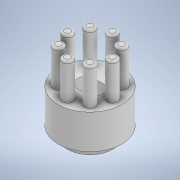
# Autodesk Inventor part: TT motor  attach to linear motion gear adapter
Saved by Autodesk Inventor 2022 (Build 260153000, 153)
## iProperties
Created: 2021-10-31
Part Number: TT motor  attach to linear motion gear adapter
Material: Generic
Document SubType Name: Modeling
Designer: alecw
Density: 1 g/cm^3
Appearance: Default
Author: alecw
Autodesk Inventor part; units mm, degrees
ref_plane "YZ Plane" through (0, 0, 0) normal (1, 0, 0) x (0, 1, 0)
ref_plane "XZ Plane" through (0, 0, 0) normal (0, 1, 0) x (-1, 0, 0)
ref_plane "XY Plane" through (0, 0, 0) normal (0, 0, 1) x (1, 0, 0)
sketch "Sketch1" plane through (0, 0, 0) normal (0, 1, 0) x (-1, 0, 0)
  circle A0 centre (0, 0) radius 2.5
  line L0 (0, 0) -> (0, 4.9)
  circle A1 centre (0, 4.9) radius 1.15
  circle A2 centre (0, 0) radius 2.7
  line L1 (0, 0) -> (0, 1.9)
  line L2 (0, 0) -> (0, -1.9)
  line L3 (0, 1.9) -> (-1.9183, 1.9)
  line L4 (0, -1.9) -> (-1.9183, -1.9)
  line L5 (0, -1.9) -> (1.9183, -1.9)
  line L6 (0, 1.9) -> (1.9183, 1.9)
  circle A3 centre (0, 0) radius 7
  circle A4 centre (-3.4648, 3.4648) radius 1.15
  circle A5 centre (-4.9, 0) radius 1.15
  circle A6 centre (-3.4648, -3.4648) radius 1.15
  circle A7 centre (0, -4.9) radius 1.15
  circle A8 centre (3.4648, -3.4648) radius 1.15
  circle A9 centre (4.9, 0) radius 1.15
  circle A10 centre (3.4648, 3.4648) radius 1.15
  circle A11 centre (0, 0) radius 4.9
  circle A12 centre (0, 0) radius 2.8
  line L7 (1.9183, -1.9) -> (2.0567, -1.9)
  line L8 (1.9183, 1.9) -> (2.0567, 1.9)
  line L9 (-1.9183, 1.9) -> (-2.0567, 1.9)
  line L10 (-1.9183, -1.9) -> (-2.0567, -1.9)
  point P0 (-1.6248, 1.9)
  point P1 (1.6248, 1.9)
  point P2 (1.6248, -1.9)
  point P3 (-1.6248, -1.9)
  dimension "d0" = 5
  dimension "d1" = 4.9
  dimension "d2" = 2.3
  dimension "d3" = 5.4
  dimension "d4" = 1.9
  dimension "d5" = 1.9
  dimension "d6" = 14
  dimension "d9" = 360
  dimension "d26" = 5.6
  constraints: 22 end point, 12 centre point, 8 point on circle, 6 coincident, 6 point on line, 2 horizontal, 2 parallel, 1 horizontal alignment, 1 vertical, 19 other
  measures "d0" diameter of A0
  measures "d1" distance of L0.start L0.end
  measures "d2" diameter of A1
  measures "d3" diameter of A2
  measures "d4" distance of L1.start L1.end
  measures "d5" distance of L1.start L2.end
  measures "d6" diameter of A3
  measures "d26" diameter of A12
extrude "Extrusion1" add sketch "Sketch1" along normal blind 3 contours A1 A11 L0 | A1 A11 A10 A9 A8 A7 A6 A5 A4 | L0 A11 A1 | A11 A1 | A11 A4 | A4 A11 | A11 A10 | A10 A11 | A11 A5 | A5 A11 | A11 A9 | A9 A11 | A11 A6 | A6 A11 | A11 A8 | A8 A11 | A11 A7 | A7 A11 | A3
extrude "Extrusion2" add sketch "Sketch1" along normal blind 6.5 from surface at 3 contours L6 L0 A0 | A0 L0 A2 L6 | L5 A2 L4 A0 | A0 L4 L5 | L0 L3 A0 | A0 L3 A2 L0 | A2 L0 A12 L8 | L7 A12 L10 A2 | A2 L9 A12 L0 | A1 A11 L0 | A1 A11 A10 A9 A8 A7 A6 A5 A4 | L0 A11 A1 | A11 A1 | A11 A4 | A4 A11 | A11 A10 | A10 A11 | A11 A5 | A5 A11 | A11 A9 | A9 A11 | A11 A6 | A6 A11 | A11 A8 | A8 A11 | A11 A7 | A7 A11 | A3
extrude "Extrusion3" add sketch "Sketch1" along normal blind 8 from surface at 9.5 contours A1 A11 L0 | L0 A11 A1 | A11 A1 | A11 A4 | A4 A11 | A11 A10 | A10 A11 | A11 A5 | A5 A11 | A11 A9 | A9 A11 | A11 A6 | A6 A11 | A11 A8 | A8 A11 | A11 A7 | A7 A11
fillet "Fillet1" radius 0.5 8 edges at (-3.75, 17.5, 0) (-2.3148, 17.5, -3.4648) (1.15, 17.5, -4.9) (4.6148, 17.5, -3.4648) (4.6148, 17.5, 3.4648) (6.05, 17.5, 0) (1.15, 17.5, 4.9) (-2.3148, 17.5, 3.4648)
chamfer "Chamfer1" distance 2 angle 45 1 edges at (7, 0, 0)
extrude "Extrusion4" add sketch "Sketch1" against normal blind 1 from surface at 3 contours L6 L0 A0 | A0 L0 A2 L6 | L5 A2 L4 A0 | A0 L4 L5 | L0 L3 A0 | A0 L3 A2 L0
chamfer "Chamfer2" distance 0.65 angle 45 2 edges at (0, 2, 1.9) (0, 2, -1.9)
body "Solid1"
